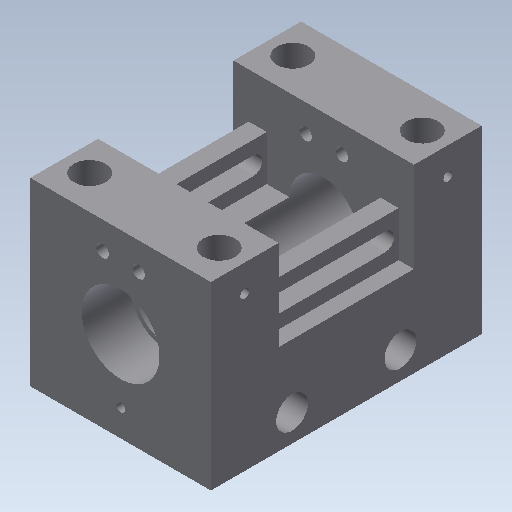
# Autodesk Inventor part: block
Saved by Autodesk Inventor 2020 (Build 240168000, 168)
## iProperties
Created: 2015-02-04
Part Number: block
Material: Generic
Document SubType Name: Modeling
Designer: Pascal
Density: 1 g/cm^3
Appearance: Default
Mass: 14.0113 g
Surface Area: 85.983 cm^2
Volume: 14.0113 cm^3
Author: Pascal
Autodesk Inventor part; units mm, degrees
ref_plane "YZ Plane" through (0, 0, 0) normal (1, 0, 0) x (0, 1, 0)
ref_plane "XZ Plane" through (0, 0, 0) normal (0, 1, 0) x (-1, 0, 0)
ref_plane "XY Plane" through (0, 0, 0) normal (0, 0, 1) x (1, 0, 0)
sketch "Sketch1" plane through (0, 0, 0) normal (0, 1, 0) x (-1, 0, 0)
  line L0 (12.0494, 19.3254) -> (-13.3506, 19.3254)
  line L1 (-13.3506, 19.3254) -> (-13.3506, -18.7746)
  line L2 (-13.3506, -18.7746) -> (12.0494, -18.7746)
  line L3 (12.0494, -18.7746) -> (12.0494, 19.3254)
  point P0 (0, 0)
  dimension "d0" = 25.4
  dimension "d1" = 38.1
  constraints: 8 end point, 2 parallel, 1 horizontal, 1 perpendicular
  measures "d0" distance of L1.end L2.end
  measures "d1" distance of L2.end L0.start
extrude "Extrusion1" add sketch "Sketch1" along normal blind 25.4
hole "Hole2" at (0.6506, 12.7, 19.3254) direction (0, 0, -1) diameter 9.652 depth 38.1
hole "Hole3" at (0.6506, 12.7, 19.3254) direction (0, 0, -1) diameter 10.9474 depth 6.731
sketch "Sketch2" plane through (0, 25.4, 0) normal (0, 1, 0) x (1, 0, 0)
  line L0 (-12.0494, 9.2496) -> (13.3506, 9.2496)
  line L1 (13.3506, 9.2496) -> (13.3506, -9.8004)
  line L2 (13.3506, -9.8004) -> (-12.0494, -9.8004)
  line L3 (-12.0494, -9.8004) -> (-12.0494, 9.2496)
  line L4 (13.3506, 18.7746) -> (-12.0494, 18.7746) projected
  line L5 (13.3506, -19.3254) -> (13.3506, 18.7746) projected
  point P0 (0, 0)
  dimension "d34" = 25.4
  dimension "d35" = 19.05
  dimension "d36" = 9.525
  constraints: 8 end point, 2 parallel, 1 horizontal, 1 perpendicular
  measures "d34" distance of L0.start L0.end
  measures "d35" distance of L0.end L1.end
  measures "d36" distance between parallel lines of L0 L4
extrude "Extrusion2" cut sketch "Sketch2" against normal blind 12.7
hole "Hole4" at (9.7629, 25.4, 14.5629) direction (0, -1, 0) diameter 4.4958 depth 25.4 clearance for "Flat Head Machine Screw (82)" size "#8" standard "Ansi Unified Screw Threads"
hole "Hole5" at (-8.4616, 25.4, 14.5629) direction (0, -1, 0) diameter 4.4958 depth 25.4 clearance for "Flat Head Machine Screw (82)" size "#8" standard "Ansi Unified Screw Threads"
hole "Hole6" at (-8.4616, 25.4, -14.0121) direction (0, -1, 0) diameter 4.4958 depth 25.4 clearance for "Flat Head Machine Screw (82)" size "#8" standard "Ansi Unified Screw Threads"
hole "Hole7" at (9.7629, 25.4, -14.0121) direction (0, -1, 0) diameter 4.4958 depth 25.4 clearance for "Flat Head Machine Screw (82)" size "#8" standard "Ansi Unified Screw Threads"
hole "Hole8" at (3.1906, 21.59, -18.7746) direction (0, 0, 1) diameter 1.778 depth 9.525 clearance for "Flat Head Machine Screw (82)" size "#0" standard "Ansi Unified Screw Threads"
hole "Hole9" at (-1.8894, 21.59, -18.7746) direction (0, 0, 1) diameter 1.778 depth 9.525 clearance for "Flat Head Machine Screw (82)" size "#0" standard "Ansi Unified Screw Threads"
hole "Hole10" at (3.1906, 21.59, 19.3254) direction (0, 0, -1) diameter 1.778 depth 9.525 clearance for "Flat Head Machine Screw (82)" size "#0" standard "Ansi Unified Screw Threads"
hole "Hole11" at (-1.8894, 21.59, 19.3254) direction (0, 0, -1) diameter 1.778 depth 9.525 tip angle 118 clearance for "Flat Head Machine Screw (82)" size "#0" standard "Ansi Unified Screw Threads"
hole "Hole14" at (13.3506, 3.81, 7.8954) direction (-1, 0, 0) diameter 4.4958 depth 25.4 clearance for "Flat Head Machine Screw (82)" size "#8" standard "Ansi Unified Screw Threads"
hole "Hole15" at (13.3506, 3.81, -7.3446) direction (-1, 0, 0) diameter 4.4958 depth 25.4 clearance for "Flat Head Machine Screw (82)" size "#8" standard "Ansi Unified Screw Threads"
sketch "Sketch6" plane through (0, 12.7, 0) normal (0, 1, 0) x (1, 0, 0)
  line L0 (8.6516, -9.8004) -> (11.1916, -9.8004)
  line L1 (11.1916, -9.8004) -> (11.1916, 9.2496)
  line L2 (11.1916, 9.2496) -> (8.6516, 9.2496)
  line L3 (8.6516, 9.2496) -> (8.6516, -9.8004)
  line L4 (13.3506, -9.8004) -> (-12.0494, -9.8004) projected
  line L5 (-12.0494, 9.2496) -> (13.3506, 9.2496) projected
  line L6 (5.4766, -9.8004) -> (5.4766, 9.2496) projected
  line L7 (13.3506, 9.2496) -> (13.3506, -9.8004) projected
  line L8 (-9.8904, -9.8004) -> (-7.3504, -9.8004)
  line L9 (-7.3504, -9.8004) -> (-7.3504, 9.2496)
  line L10 (-7.3504, 9.2496) -> (-9.8904, 9.2496)
  line L11 (-9.8904, 9.2496) -> (-9.8904, -9.8004)
  line L12 (-4.1754, 9.2496) -> (-4.1754, -9.8004) projected
  line L13 (-12.0494, -9.8004) -> (-12.0494, 9.2496) projected
  point P0 (0, 0)
  dimension "d179" = 0
  dimension "d180" = 0
  dimension "d181" = 2.54
  dimension "d182" = 3.175
  dimension "d183" = 2.159
  dimension "d184" = 0
  dimension "d185" = 0
  dimension "d186" = 3.175
  dimension "d187" = 2.54
  dimension "d188" = 2.159
  constraints: 16 end point, 4 parallel, 2 horizontal, 2 perpendicular
  measures "d179" distance between parallel lines of L4 L0
  measures "d180" distance between parallel lines of L5 L2
  measures "d181" distance between parallel lines of L1 L3
  measures "d182" distance between parallel lines of L6 L3
  measures "d183" distance between parallel lines of L7 L1
  measures "d184" distance between parallel lines of L5 L10
  measures "d185" distance between parallel lines of L4 L8
  measures "d186" distance between parallel lines of L12 L9
  measures "d187" distance between parallel lines of L11 L9
  measures "d188" distance between parallel lines of L13 L11
extrude "Extrusion4" add sketch "Sketch6" along normal blind 6.35 contours L3 L2 L1 L0 | L4 L11 L5 L9
sketch "Sketch7" plane through (11.1916, 12.7, 9.8004) normal (1, 0, 0) x (0, 0, -1)
  line L0 (0.635, 4.445) -> (18.415, 4.445)
  line L1 (18.415, 4.445) -> (18.415, 1.905)
  line L2 (18.415, 1.905) -> (0.635, 1.905)
  line L3 (0.635, 1.905) -> (0.635, 4.445)
  line L4 (19.05, 0) -> (0, 0) projected
  line L5 (0, 6.35) -> (19.05, 6.35) projected
  line L6 (0, 0) -> (0, 6.35) projected
  line L7 (19.05, 12.7) -> (19.05, 0) projected
  point P0 (9.8004, -12.7)
  dimension "d191" = 2.54
  dimension "d192" = 1.905
  dimension "d193" = 1.905
  dimension "d194" = 0.635
  dimension "d195" = 0.635
  constraints: 8 end point, 2 parallel, 1 horizontal, 1 perpendicular
  measures "d191" distance between parallel lines of L2 L0
  measures "d192" distance between parallel lines of L4 L2
  measures "d193" distance between parallel lines of L5 L0
  measures "d194" distance between parallel lines of L3 L6
  measures "d195" distance between parallel lines of L1 L7
extrude "Extrusion5" cut sketch "Sketch7" against normal through all contours L0 L1 L2 L3
fillet "Fillet1" radius 1.27 8 edges at (9.9216, 17.145, 9.1654) (9.9216, 14.605, 9.1654) (-8.6204, 17.145, -8.6146) (9.9216, 14.605, -8.6146) (9.9216, 17.145, -8.6146) (-8.6204, 14.605, -8.6146) (-8.6204, 14.605, 9.1654) (-8.6204, 17.145, 9.1654)
hole "Hole16" at (13.3506, 21.59, 14.5629) direction (-1, 0, 0) diameter 1.27 end through all
hole "Hole17" at (13.3506, 21.59, -14.0121) direction (-1, 0, 0) diameter 1.27 end through all
hole "Hole18" at (0.6506, 3.81, -18.7746) direction (0, 0, 1) diameter 1.27 end through all
body "Solid1"
